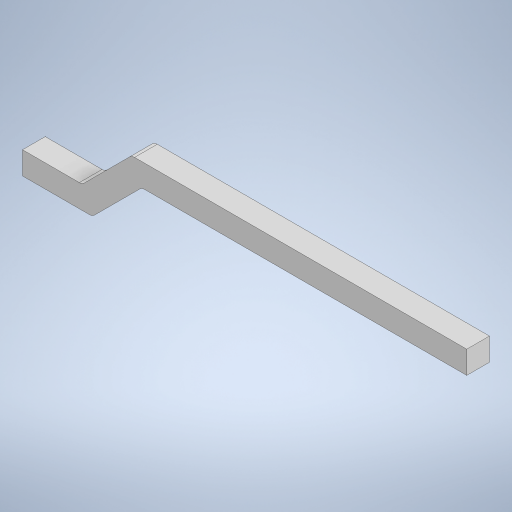
# Autodesk Inventor part: Pin
Saved by Autodesk Inventor 2023 (Build 270158000, 158)
## iProperties
Created: 2023-01-17
Part Number: Pin
Material: Generisch
Document SubType Name: Sheet Metal
Designer: remoh
Density: 1 g/cm^3
Sheet Metal Rule: Standard_mm
Appearance: Vorgabe
Author: remoh
Autodesk Inventor part; units mm, degrees
ref_plane "YZ Plane" through (0, 0, 0) normal (1, 0, 0) x (0, 1, 0)
ref_plane "XZ Plane" through (0, 0, 0) normal (0, 1, 0) x (-1, 0, 0)
ref_plane "XY Plane" through (0, 0, 0) normal (0, 0, 1) x (1, 0, 0)
sketch "Skizze1" plane through (0, 0, 0) normal (0, 0, 1) x (1, 0, 0)
  line L0 (0, 0) -> (2, 0)
  line L1 (2, 0) -> (3.4142, 1.4142)
  line L2 (3.4142, 1.4142) -> (12.7142, 1.4142)
  line L3 (12.7142, 1.4142) -> (12.7142, 2.0642)
  line L4 (12.7142, 2.0642) -> (3.1238, 2.0642)
  line L5 (3.1238, 2.0642) -> (1.7095, 0.65)
  line L6 (1.7095, 0.65) -> (0, 0.65)
  line L7 (0, 0.65) -> (0, 0)
  dimension "d0" = 2
  dimension "d1" = 2
  dimension "d2" = 9.3
  dimension "d3" = 0.65
  dimension "d4" = 0.65
  dimension "d5" = 135
  dimension "d6" = 0.665
  constraints: 16 end point, 3 parallel, 3 perpendicular, 1 horizontal
  measures "d0" distance of L0.start L0.end
  measures "d1" distance of L0.end L1.end
  measures "d2" distance of L1.end L2.end
  measures "d3" distance of L2.end L3.end
  measures "d4" distance of L6.end L0.start
  measures "d5" angle of L1 L0
  measures "d6" distance between parallel lines of L1 L5
extrude "Extrusion1" add sketch "Skizze1" along normal blind 0.65
fillet "Rundung1" radius 0.2 4 edges at (2, 0, 0.325) (1.7095, 0.65, 0.325) (3.1238, 2.0642, 0.325) (3.4142, 1.4142, 0.325)
equation "\"Biegeradius\" = Stärke"
equation "\"BreiteBiegungsfreistellung\" = Stärke"
equation "\"TiefeBiegungsfreistellung\" = 0.5 * Stärke"
equation "\"GrößeEckenfreistellung\" = 4 * Stärke"
equation "\"MinimalRest\" = 2 * Stärke"
equation "\"Übergangsradius\" = Biegeradius"
equation "\"JacobiRadiusGröße\" = Biegeradius"
equation "\"Abstandsgröße\" = Stärke"
equation "\"Stärke\" = 0.5"
